Autodesk Fusion 360 part; units mm, degrees
(part 2 of 2)
  spline S387 degree 3 poles (34.5927, -13.5913) (34.3582, -13.7521) (34.3613, -14.0864) (34.6169, -14.2051) knots 0 0 0 0 1 1 1 1
  spline S388 degree 3 poles (34.6169, -14.2051) (34.8301, -14.3042) (35.0655, -14.3616) (35.2961, -14.416) knots 0 0 0 0 1 1 1 1
  spline S389 degree 3 poles (35.2961, -14.416) (35.7418, -14.5212) (36.1929, -14.6061) (36.6092, -14.8078) knots 0 0 0 0 1 1 1 1
  spline S390 degree 3 poles (36.6092, -14.8078) (37.0095, -15.0019) (37.3295, -15.2758) (37.4532, -15.7221) knots 0 0 0 0 1 1 1 1
  spline S391 degree 3 poles (37.4532, -15.7221) (37.6514, -16.4372) (37.453, -17.5153) (36.2859, -17.8987) knots 0 0 0 0 1 1 1 1
  spline S392 degree 3 poles (36.2859, -17.8987) (36.0122, -17.9886) (35.7152, -18.0078) (35.4182, -18.0602) knots 0 0 0 0 1 1 1 1
  spline S393 degree 3 poles (1.7611, -15.7325) (1.6566, -15.083) (1.7044, -14.4582) (1.9794, -13.8657) knots 0 0 0 0 1 1 1 1
  spline S394 degree 3 poles (1.9794, -13.8657) (2.4019, -12.9553) (3.1324, -12.4438) (4.1098, -12.2797) knots 0 0 0 0 1 1 1 1
  spline S395 degree 3 poles (4.1098, -12.2797) (4.7174, -12.1777) (5.3126, -12.2327) (5.874, -12.507) knots 0 0 0 0 1 1 1 1
  spline S396 degree 3 poles (5.874, -12.507) (6.4138, -12.7708) (6.7834, -13.1999) (7.0529, -13.7428) knots 0 0 0 0 1 1 1 1
  spline S397 degree 3 poles (7.0529, -13.7428) (6.6476, -13.9409) (6.2483, -14.1361) (5.8446, -14.3334) knots 0 0 0 0 1 1 1 1
  spline S398 degree 3 poles (5.8446, -14.3334) (5.6784, -13.9656) (5.4119, -13.709) (5.0331, -13.581) knots 0 0 0 0 1 1 1 1
  spline S399 degree 3 poles (5.0331, -13.581) (4.4189, -13.3734) (3.7265, -13.6377) (3.3907, -14.2271) knots 0 0 0 0 1 1 1 1
  spline S400 degree 3 poles (3.3907, -14.2271) (3.0448, -14.8341) (3.0431, -15.461) (3.3893, -16.0671) knots 0 0 0 0 1 1 1 1
  spline S401 degree 3 poles (3.3893, -16.0671) (3.665, -16.5497) (4.104, -16.799) (4.6612, -16.7813) knots 0 0 0 0 1 1 1 1
  spline S402 degree 3 poles (4.6612, -16.7813) (5.2156, -16.7636) (5.6028, -16.4677) (5.8469, -15.9661) knots 0 0 0 0 1 1 1 1
  spline S403 degree 3 poles (5.8469, -15.9661) (6.2462, -16.1611) (6.6455, -16.3561) (7.0532, -16.5552) knots 0 0 0 0 1 1 1 1
  spline S404 degree 3 poles (7.0532, -16.5552) (6.7147, -17.2311) (6.2227, -17.719) (5.4961, -17.9369) knots 0 0 0 0 1 1 1 1
  spline S405 degree 3 poles (5.4961, -17.9369) (4.3949, -18.2671) (3.0452, -17.956) (2.2925, -16.9597) knots 0 0 0 0 1 1 1 1
  spline S406 degree 3 poles (2.2925, -16.9597) (2.0179, -16.5963) (1.8461, -16.1886) (1.7611, -15.7325) knots 0 0 0 0 1 1 1 1
  spline S407 degree 3 poles (29.4232, -16.6466) (28.9989, -16.6687) (28.5839, -16.6888) (28.1623, -16.7091) knots 0 0 0 0 1 1 1 1
  spline S408 degree 3 poles (28.1623, -16.7091) (28.1623, -15.6542) (28.1623, -14.6276) (28.1623, -13.6001) knots 0 0 0 0 1 1 1 1
  spline S409 degree 3 poles (28.1623, -13.6001) (28.167, -13.5963) (28.1729, -13.5875) (28.1786, -13.5876) knots 0 0 0 0 1 1 1 1
  spline S410 degree 3 poles (28.1786, -13.5876) (28.5349, -13.5912) (28.8922, -13.5806) (29.2473, -13.6029) knots 0 0 0 0 1 1 1 1
  spline S411 degree 3 poles (29.2473, -13.6029) (29.9248, -13.6453) (30.4264, -14.1244) (30.5242, -14.7949) knots 0 0 0 0 1 1 1 1
  spline S412 degree 3 poles (30.5242, -14.7949) (30.5663, -15.0838) (30.5647, -15.3705) (30.4751, -15.6498) knots 0 0 0 0 1 1 1 1
  spline S413 degree 3 poles (30.4751, -15.6498) (30.3086, -16.1687) (29.9645, -16.5062) (29.4232, -16.6466) knots 0 0 0 0 1 1 1 1
  spline S414 degree 3 poles (23.9741, -14.7295) (23.8494, -14.7585) (23.7324, -14.8009) (23.6144, -14.804) knots 0 0 0 0 1 1 1 1
  spline S415 degree 3 poles (23.6144, -14.804) (23.2583, -14.8134) (22.9018, -14.8074) (22.5377, -14.8074) knots 0 0 0 0 1 1 1 1
  spline S416 degree 3 poles (22.5377, -14.8074) (22.5377, -14.3901) (22.5377, -13.9753) (22.5377, -13.5469) knots 0 0 0 0 1 1 1 1
  spline S417 degree 3 poles (22.5377, -13.5469) (22.6439, -13.5469) (22.7521, -13.5462) (22.8603, -13.547) knots 0 0 0 0 1 1 1 1
  spline S418 degree 3 poles (22.8603, -13.547) (23.1484, -13.549) (23.437, -13.543) (23.7247, -13.5566) knots 0 0 0 0 1 1 1 1
  spline S419 degree 3 poles (23.7247, -13.5566) (23.9952, -13.5694) (24.2146, -13.754) (24.2836, -13.9997) knots 0 0 0 0 1 1 1 1
  spline S420 degree 3 poles (24.2836, -13.9997) (24.3663, -14.2948) (24.2534, -14.5657) (23.9741, -14.7295) knots 0 0 0 0 1 1 1 1
  spline S421 degree 3 poles (17.4059, -16.7681) (16.6257, -16.8897) (15.9245, -16.3984) (15.7459, -15.6076) knots 0 0 0 0 1 1 1 1
  spline S422 degree 3 poles (15.7459, -15.6076) (15.6525, -15.194) (15.6748, -14.7855) (15.8437, -14.393) knots 0 0 0 0 1 1 1 1
  spline S423 degree 3 poles (15.8437, -14.393) (16.0963, -13.806) (16.6486, -13.473) (17.2886, -13.5143) knots 0 0 0 0 1 1 1 1
  spline S424 degree 3 poles (17.2886, -13.5143) (17.929, -13.5557) (18.437, -13.9655) (18.6061, -14.6024) knots 0 0 0 0 1 1 1 1
  spline S425 degree 3 poles (18.6061, -14.6024) (18.7615, -15.1877) (18.7026, -15.748) (18.3279, -16.2445) knots 0 0 0 0 1 1 1 1
  spline S426 degree 3 poles (18.3279, -16.2445) (18.101, -16.5451) (17.7911, -16.7171) (17.4059, -16.7681) knots 0 0 0 0 1 1 1 1
  line L0 (0.0228, -0.0228) -> (39.98, -0.0228)
  line L1 (39.98, -0.0228) -> (39.98, -30.2754)
  line L2 (39.98, -30.2754) -> (0.0228, -30.2754)
  line L3 (0.0228, -30.2754) -> (0.0228, -0.0228)
  constraint horizontal L0
  constraint vertical L1
  constraint horizontal L2
  constraint vertical L3
  constraint coincident S2.end S3.start
  constraint coincident S0.end S1.start
sketch "Sketch2" plane through (0, 0, 0) normal (0, 0, 1) x (1, 0, 0)
  line L0 (0, 0) -> (40, 0)
  line L1 (40, 0) -> (40, -30.3)
  line L2 (40, -30.3) -> (0, -30.3)
  line L3 (0, -30.3) -> (0, 0)
  constraint horizontal L0
  constraint vertical L1
  constraint horizontal L2
  constraint vertical L3
  constraint coincident L0.start L3.end
extrude "Extrude1" add sketch "Sketch2" along normal blind 4
extrude "Extrude2" cut sketch "Sketch1" against normal blind 1 from surface at 4 contours S5 S6 S7 S8 S9 S10 S11 S196 S197 S198 S199 S200 S201 S202 | S12 S13 S14 S15 S16 S17 S18 S203 S204 S205 S206 S207 S208 S209 | S19 S20 S21 S22 S23 S24 S25 S210 S211 S212 S213 S214 S215 S216 | S26 S27 S28 S29 S30 S31 S32 S217 S218 S219 S220 S221 S222 S223 | S33 S34 S35 S36 S37 S38 S39 S224 S225 S226 S227 S228 S229 S230 | S40 S41 S42 S43 S44 S45 S46 S231 S232 S233 S234 S235 S236 S237 | S47 S48 S49 S50 S51 S52 S53 S238 S239 S240 S241 S242 S243 S244 | S54 S55 S56 S57 S58 S59 S60 S245 S246 S247 S248 S249 S250 S251 | S61 S62 S63 S64 S65 S66 S67 S68 S69 S70 S252 S253 S254 S255 S256 S257 S258 S259 S260 S261 | S71 S72 S73 S74 S75 S76 S77 S78 S79 S262 S263 S264 S265 S266 S267 S268 S269 S270 | S80 S81 S82 S83 S84 S85 S86 S87 S88 S271 S272 S273 S274 S275 S276 S277 S278 S279 | S89 S90 S91 S92 S93 S94 S95 S96 S97 S280 S281 S282 S283 S284 S285 S286 S287 S288 | S98 S99 S100 S101 S102 S103 S104 S105 S106 S289 S290 S291 S292 S293 S294 S295 S296 S297 | S107 S108 S109 S110 S111 S112 S113 S114 S115 S298 S299 S300 S301 S302 S303 S304 S305 S306 | S116 S117 S118 S119 S120 S121 S122 S123 S124 S307 S308 S309 S310 S311 S312 S313 S314 S315 | S125 S126 S127 S128 S129 S130 S131 S132 S133 S134 S135 S136 S323 S324 S325 S326 S327 S328 S329 S330 S331 S332 S333 S334 | S137 S138 S139 S140 S141 S142 S143 S144 S342 S343 S344 S345 S346 S347 S348 S349 | S145 S146 S147 S148 S149 S150 S151 S152 S153 S154 S155 S156 S157 S356 S357 S358 S359 S360 S361 S362 S363 S364 S365 S366 S367 S368 | S158 S159 S160 S161 S162 S163 S164 S165 S166 S167 S168 S169 S170 S171 S172 S173 S174 S175 S176 S177 S178 S179 S180 S181 S369 S370 S371 S372 S373 S374 S375 S376 S377 S378 S379 S380 S381 S382 S383 S384 S385 S386 S387 S388 S389 S390 S391 S392 | S182 S183 S184 S185 S186 S187 S188 S189 S190 S191 S192 S193 S194 S195 S393 S394 S395 S396 S397 S398 S399 S400 S401 S402 S403 S404 S405 S406
